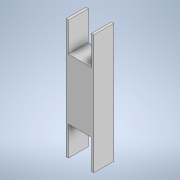
# Autodesk Inventor part: armj3
Saved by Autodesk Inventor 2020 (Build 240168000, 168)
## iProperties
Created: 2021-03-31
Part Number: armj3
Material: Generic
Document SubType Name: Modeling
Designer: super
Density: 1 g/cm^3
Appearance: Default
Mass: 312.24 g
Surface Area: 1079.2 cm^2
Volume: 312.24 cm^3
Author: super
Autodesk Inventor part; units mm, degrees
ref_plane "YZ Plane" through (0, 0, 0) normal (1, 0, 0) x (0, 1, 0)
ref_plane "XZ Plane" through (0, 0, 0) normal (0, 1, 0) x (-1, 0, 0)
ref_plane "XY Plane" through (0, 0, 0) normal (0, 0, 1) x (1, 0, 0)
sketch "Sketch1" plane through (0, 0, 0) normal (0, 0, 1) x (1, 0, 0)
  line L0 (0, 80) -> (0, 0)
  line L1 (0, 0) -> (70, 0)
  line L2 (70, 0) -> (70, 80)
  line L3 (6, 80) -> (6, 6)
  line L4 (6, 6) -> (64, 6)
  line L5 (64, 6) -> (64, 80)
  line L6 (0, 80) -> (6, 80)
  line L7 (64, 80) -> (70, 80)
  line L8 (0, -70) -> (70, -70)
  line L9 (0, -220) -> (0, -140)
  line L10 (0, -140) -> (70, -140)
  line L11 (70, -140) -> (70, -220)
  line L12 (6, -220) -> (6, -146)
  line L13 (6, -146) -> (64, -146)
  line L14 (64, -146) -> (64, -220)
  line L15 (0, -220) -> (6, -220)
  line L16 (64, -220) -> (70, -220)
  dimension "d0" = 70
  dimension "d1" = 80
  dimension "d2" = 80
  dimension "d3" = 6
  dimension "d10" = 70
  constraints: 34 end point, 8 symmetric about line, 3 horizontal, 3 perpendicular, 1 vertical, 2 other
  measures "d0" distance of L0.end L1.end
  measures "d1" distance of L1.end L2.end
  measures "d2" distance of L0.start L0.end
  measures "d3" distance between parallel lines of L0 L3
  measures "d10" distance of L8.start L0.end
extrude "Extrusion1" add sketch "Sketch1" along normal blind 50
sketch "Sketch2" plane through (0, 0, 0) normal (0, -1, 0) x (1, 0, 0)
  line L0 (6, 0) -> (0, 0) projected
  line L1 (0, 50) -> (70, 50) projected
  line L2 (0, 0) -> (70, 0)
  line L3 (70, 0) -> (70, 50)
  line L4 (70, 50) -> (0, 50)
  line L5 (0, 50) -> (0, 0)
  line L6 (6, 6) -> (64, 6)
  line L7 (64, 6) -> (64, 44)
  line L8 (64, 44) -> (6, 44)
  line L9 (6, 44) -> (6, 6)
  dimension "d7" = 6
  constraints: 16 end point, 4 parallel, 2 perpendicular, 1 horizontal, 3 other
  measures "d7" distance between parallel lines of L5 L9
extrude "Extrusion2" add sketch "Sketch2" along normal blind 140
body "Solid1"
